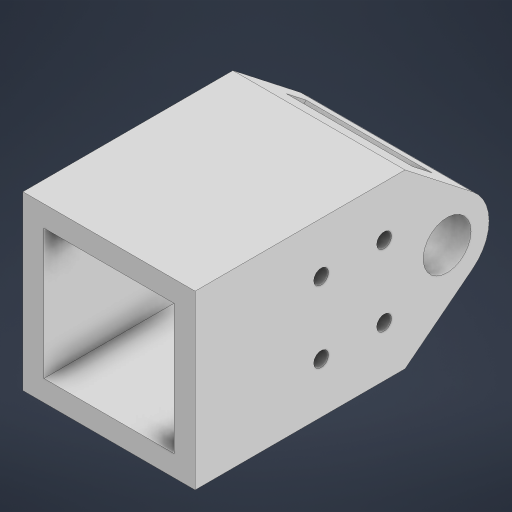
# Autodesk Inventor part: CS_Climb_Outer_Tube_End_Cap
Saved by Autodesk Inventor 2023 (Build 270158000, 158)
## iProperties
Created: 2024-02-19
Part Number: CS_Climb_Outer_Tube_End_Cap
Material: Generic
Document SubType Name: Modeling
Designer: kelle
Density: 1 g/cm^3
Appearance: Default
Author: kelle
Autodesk Inventor part; units mm, degrees
ref_plane "YZ Plane" through (0, 0, 0) normal (1, 0, 0) x (0, 1, 0)
ref_plane "XZ Plane" through (0, 0, 0) normal (0, 1, 0) x (-1, 0, 0)
ref_plane "XY Plane" through (0, 0, 0) normal (0, 0, 1) x (1, 0, 0)
sketch "Sketch1" plane through (0, 0, 0) normal (0, 0, 1) x (1, 0, 0)
  line L0 (19.685, -19.685) -> (-19.685, -19.685)
  line L1 (-19.685, -19.685) -> (-19.685, 19.685)
  line L2 (-19.685, 19.685) -> (19.685, 19.685)
  line L3 (19.685, 19.685) -> (19.685, -19.685)
  line L4 (19.685, -19.685) -> (-19.685, 19.685) construction
  line L5 (-19.685, -19.685) -> (19.685, 19.685) construction
  line L6 (26.035, 26.035) -> (-26.035, 26.035)
  line L7 (-26.035, 26.035) -> (-26.035, -26.035)
  line L8 (-26.035, -26.035) -> (26.035, -26.035)
  line L9 (26.035, -26.035) -> (26.035, 26.035)
  point P0 (0, 0)
  dimension "d0" = 39.37
  dimension "d1" = 39.37
  dimension "d2" = 6.35
  constraints: 20 end point, 4 parallel, 2 midpoint, 2 perpendicular, 1 horizontal, 3 other
  measures "d0" distance of L1.end L2.end
  measures "d1" distance of L0.end L1.end
  measures "d2" distance between parallel lines of L2 L6
extrude "Extrusion1" add sketch "Sketch1" along normal blind 63.5
sketch "Sketch2" plane through (26.035, -26.035, 0) normal (1, 0, 0) x (0, 0, -1)
  line L0 (-63.5, 45.72) -> (-63.5, 6.35) construction
  line L1 (-63.5, 26.035) -> (50.8, 26.035) construction
  circle A0 centre (12.7, 26.035) radius 7.25
  line L2 (0, 0) -> (0, 52.07) projected
  circle A1 centre (12.7, 26.035) radius 12.7
  line L3 (0, 52.07) -> (-63.5, 52.07) projected
  line L4 (0, 52.07) -> (20.5177, 36.0436)
  line L5 (0, 0) -> (-63.5, 0) projected
  line L6 (0, 0) -> (20.5177, 16.0264)
  point P0 (0, 26.035)
  dimension "d5" = 114.3
  dimension "d6" = 14.5
  dimension "d7" = 12.7
  dimension "d8" = 25.4
  constraints: 6 end point, 2 centre point, 2 point on circle, 2 tangent, 1 coincident, 1 horizontal, 1 midpoint, 1 point on line
  measures "d5" distance of L1.start L1.end
  measures "d6" diameter of A0
  measures "d7" distance from line of L2 A0.centre
  measures "d8" diameter of A1
extrude "Extrusion2" add sketch "Sketch2" against normal up to surface (52.07 mm away)
sketch "Sketch3" plane through (26.035, -26.035, 63.5) normal (1, 0, 0) x (0, 0, -1)
  circle A0 centre (76.2, 26.035) radius 7.25 projected
  line L0 (63.5, 52.07) -> (0, 52.07) projected
  line L1 (0, 0) -> (0, 52.07) projected
  line L2 (63.5, 0) -> (0, 0) projected
  line L3 (63.5, 0) -> (84.0177, 16.0264) projected
  arc A1 (84.0177, 16.0264) -> (84.0177, 36.0436) centre (76.2, 26.035) ccw projected
  line L4 (84.0177, 36.0436) -> (63.5, 52.07) projected
  line L5 (63.5, 45.72) -> (63.5, 6.35) construction
  circle A2 centre (57.15, 36.83) radius 2.25
  line L6 (63.5, 45.72) -> (0, 45.72) construction
  line L7 (63.5, 45.72) -> (0, 45.72) construction
  line L8 (63.5, 6.35) -> (0, 6.35) construction
  line L9 (63.5, 6.35) -> (0, 6.35) construction
  circle A3 centre (57.15, 15.24) radius 2.25
  circle A4 centre (38.1, 36.83) radius 2.25
  circle A5 centre (38.1, 15.24) radius 2.25
  point P0 (63.5, 26.035)
  dimension "d11" = 4.5
  dimension "d12" = 6.35
  dimension "d13" = 8.89
  dimension "d14" = 4.5
  dimension "d15" = 6.35
  dimension "d16" = 8.89
  dimension "d17" = 4.5
  dimension "d18" = 19.05
  dimension "d19" = 8.89
  dimension "d20" = 4.5
  dimension "d21" = 19.05
  dimension "d22" = 8.89
  constraints: 4 centre point, 4 end point, 1 collinear
  measures "d11" diameter of A2
  measures "d12" distance from line of L5 A2.centre
  measures "d13" distance from line of L6 A2.centre
  measures "d14" diameter of A3
  measures "d15" distance from line of L5 A3.centre
  measures "d16" distance from line of L8 A3.centre
  measures "d17" diameter of A4
  measures "d18" distance of A2.centre A4.centre
  measures "d19" distance from line of L6 A4.centre
  measures "d20" diameter of A5
  measures "d21" distance of A3.centre A5.centre
  measures "d22" distance from line of L8 A5.centre
extrude "Extrusion3" cut sketch "Sketch3" against normal through all contours A2 | A3 | A4 | A5
sketch "Sketch5" plane through (-26.035, 26.035, 0) normal (0, 0.7880827, -0.6155694) x (1, 0, 0)
  line L0 (0, 26.035) -> (0, 0) projected
  line L1 (52.07, 0) -> (0, 0) projected
  line L2 (52.07, 26.035) -> (52.07, 0) projected
  line L3 (52.07, 26.035) -> (0, 26.035) projected
  line L4 (6.35, 3.9089) -> (45.72, 3.9089) construction
  line L5 (26.035, 3.9089) -> (26.035, 26.035) construction
  line L6 (6.35, 15.4171) -> (0, 15.4171) construction
  line L7 (0, 15.4171) -> (52.07, 15.4171) construction
  line L8 (52.07, 15.4171) -> (45.72, 15.4171) construction
  line L9 (45.085, 19.1671) -> (6.985, 19.1671)
  line L10 (6.985, 19.1671) -> (6.985, 11.6671)
  line L11 (6.985, 11.6671) -> (45.085, 11.6671)
  line L12 (45.085, 11.6671) -> (45.085, 19.1671)
  line L13 (45.085, 19.1671) -> (6.985, 11.6671) construction
  line L14 (6.985, 19.1671) -> (45.085, 11.6671) construction
  point P0 (26.035, 16.0264)
  point P1 (26.035, 15.4171)
  dimension "d30" = 38.1
  dimension "d31" = 7.5
  constraints: 16 end point, 5 midpoint, 4 point on line, 2 parallel, 1 horizontal, 1 perpendicular
  measures "d30" distance of L11.end L10.end
  measures "d31" distance of L10.end L9.end
extrude "Extrusion5" cut sketch "Sketch5" against normal up to surface contours L12 L11 L10 L9 surface through (19.685, -19.685, 0) normal (0, 1, 0)
body "Solid1"
